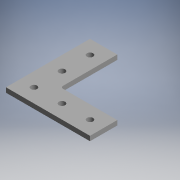
# Autodesk Inventor part: 4481
Saved by Autodesk Inventor 2017.3 (Build 213256000, 256)
## iProperties
Part Number: 4481
Material: Generic
Catalog Web Link: www.cadenas.de
Description: 4081, 4481, 4081-Black, 4481-Black-Joining Plates - 5 Hole "L" Joining Plate
Vendor: 8020
Document SubType Name: Modeling
Designer: partserver
Manufacturer: 8020
Mass: 43.3818 g
Surface Area: 173.891 cm^2
Volume: 43.3818 cm^3
Density: 1 g/cm^3
Appearance: PSOLRGB-191-191-191
Category: PARTsolutions
Company: 8020
Title: 4481
Author: Cadenas PARTsolutions
Comments: Joining Plates - 5 Hole "L" Joining Plate
PSOL_IDENT_0: {$CADENAS_DATA\23d-libs\8020\inch\joining_plates\4081.prj},176 {VTYP=3D},{NB=4481},{LINA=4481},{NN=4
PSOL_IDENT_1: 081, 4481, 4081-Black, 4481-Black},{DATE=31.07.2020 09:21:18},{GEOMDATE=19.07.2017 15:57:14},{VERSIO
PSOL_IDENT_2: N=},{LINEID=30},{WBVAR=},{WBNUMERIC=}  {NB=4481},{LINA=4481},{KT=DUMMY},{PN=4481},{A=0.750},{B=1.500
PSOL_IDENT_3: },{C=1.460},{D=1.460},{E=4.5000},{F=0.328},{G=0.125},{T=0.250},{W=.296},{COLOR=.75,.75,.75}
NB: 4481
NN: 4081, 4481, 4081-Black, 4481-Black
NT: Joining Plates - 5 Hole "L" Joining Plate
NBSYN: $PN.
LINA: 4481
CATALOG: 80/20
PN: 4481
A: 0.75
B: 1.5
C: 1.46
D: 1.46
E: 4.5
F: 0.328
G: 0.125
T: 0.25
W: .296
SUPPLIER: 8020
ARTICLENO: 4481
BOMINFO: 4481
CREATOR: CADENAS GmbH
Autodesk Inventor part; units mm, degrees
ref_plane "YZ Plane" through (0, 0, 0) normal (1, 0, 0) x (0, 1, 0)
ref_plane "XZ Plane" through (0, 0, 0) normal (0, 1, 0) x (-1, 0, 0)
ref_plane "XY Plane" through (0, 0, 0) normal (0, 0, 1) x (1, 0, 0)
sketch "Sketch_1" plane through (0, 0, 0) normal (0, 0, 1) x (1, 0, 0)
  line L0 (-114.3, 37.084) -> (-114.3, 0)
  line L1 (-114.3, 0) -> (0, 0)
  line L2 (0, 0) -> (0, 114.3)
  line L3 (0, 114.3) -> (-37.084, 114.3)
  line L4 (-37.084, 114.3) -> (-37.084, 40.259)
  arc A0 (-40.259, 37.084) -> (-37.084, 40.259) centre (-40.259, 40.259) ccw
  line L5 (-40.259, 37.084) -> (-114.3, 37.084)
  circle A1 centre (-19.05, 19.05) radius 4.1656
  circle A2 centre (-19.05, 95.25) radius 4.1656
  circle A3 centre (-19.05, 57.15) radius 4.1656
  circle A4 centre (-57.15, 19.05) radius 4.1656
  circle A5 centre (-95.25, 19.05) radius 4.1656
  constraints: 12 end point, 6 centre point, 2 point on circle
extrude "Extrusion1" add sketch "Sketch_1" along normal blind 6.35
body "Solid1"
